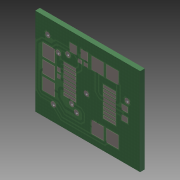
# Autodesk Inventor part: Health_module_uCBoard
Saved by Autodesk Inventor 2013 (Build 170138000, 138)
## iProperties
Created: 2015-07-04
Part Number: Health_module_uCBoard
Material: Ogólny
Document SubType Name: Modeling
Designer: terg
Density: 1 g/cm^3
Author: terg
Autodesk Inventor part; units mm, degrees
ref_plane "YZ Plane" through (0, 0, 0) normal (1, 0, 0) x (0, 1, 0)
ref_plane "XZ Plane" through (0, 0, 0) normal (0, 1, 0) x (-1, 0, 0)
ref_plane "XY Plane" through (0, 0, 0) normal (0, 0, 1) x (1, 0, 0)
sketch "Szkic1" plane through (0, 0, 0) normal (0, 1, 0) x (-1, 0, 0)
  line L0 (0, 0) -> (-18, 0)
  line L1 (-18, 0) -> (-18, -15)
  line L2 (-18, -15) -> (0, -15)
  line L3 (0, -15) -> (0, 0)
  dimension "d0" = 18
  dimension "d1" = 15
  constraints: 8 end point, 2 parallel, 1 horizontal, 1 perpendicular
  measures "d0" distance of L2.end L1.end
  measures "d1" distance of L1.end L0.end
extrude "Wyciągnięcie proste1" add sketch "Szkic1" along normal blind 0.8
sketch "Szkic2" plane through (0, 0.8, 0) normal (0, 1, 0) x (1, 0, 0)
  line L0 (0, 0) -> (18, 0) projected
  line L1 (18, 0) -> (18, 15) projected
  line L2 (18, 15) -> (0, 15) projected
  line L3 (0, 15) -> (0, 0) projected
  line L4 (0.0227, 15) -> (17.9773, 15) construction
  line L5 (17.9773, 15) -> (17.9773, 0) construction
  line L6 (17.9773, 0) -> (0.0227, 0) construction
  line L7 (0.0227, 0) -> (0.0227, 15) construction
  dimension "d9" = 0
  dimension "d10" = 0.0227
  dimension "d11" = 0
  dimension "d13" = 0.0227
  constraints: 2 other
  measures "d9" distance between parallel lines of L2 L4
  measures "d10" distance between parallel lines of L3 L7
  measures "d11" distance between parallel lines of L0 L6
  measures "d13" distance between parallel lines of L1 L5
decal "Pokrycie bitmapą1"
sketch "Szkic3" plane through (0, 0, 0) normal (0, -1, 0) x (1, 0, 0)
  line L0 (0, 0) -> (18, 0) projected
  line L1 (0, -15) -> (0, 0) projected
  line L2 (18, -15) -> (0, -15) projected
  line L3 (18, 0) -> (18, -15) projected
  line L4 (17.9962, -15) -> (0.0038, -15) construction
  line L5 (0.0038, -15) -> (0.0038, 0) construction
  line L6 (0.0038, 0) -> (17.9962, 0) construction
  line L7 (17.9962, 0) -> (17.9962, -15) construction
  dimension "d26" = 0
  dimension "d27" = 0.0038
  dimension "d28" = 0
  dimension "d29" = 0.0038
  constraints: 2 other
  measures "d26" distance between parallel lines of L2 L4
  measures "d27" distance between parallel lines of L3 L7
  measures "d28" distance between parallel lines of L0 L6
  measures "d29" distance between parallel lines of L1 L5
decal "Pokrycie bitmapą2"
sketch "Szkic4" plane through (0, 0.8, 0) normal (0, 1, 0) x (1, 0, 0)
  point P0 (3.1212, 12.4241)
  point P1 (6.264, 10.7764)
  point P2 (7.0841, 11.6729)
  point P3 (8.7816, 7.9997)
  point P4 (3.963, 4.3412)
  point P5 (5.625, 3.7513)
  point P6 (2.1559, 2.5529)
  point P7 (15.7881, 5.5924)
hole "Otwór1" at (3.1212, 0.8, -12.4241) at (6.264, 0.8, -10.7764) at (7.0841, 0.8, -11.6729) at (8.7816, 0.8, -7.9997) at (3.963, 0.8, -4.3412) at (5.625, 0.8, -3.7513) at (2.1559, 0.8, -2.5529) at (15.7881, 0.8, -5.5924) direction (0, -1, 0) diameter 0.4 depth 8
equation "\"d10\" = d13"
equation "\"d27\" = d29"
